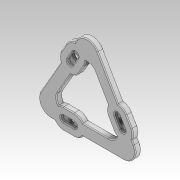
# Autodesk Inventor part: ValveThing2
Saved by Autodesk Inventor 2020 (Build 240168000, 168)
## iProperties
Created: 2022-01-09
Part Number: ValveThing2
Material: Generic
Document SubType Name: Modeling
Designer: DDeGo
Density: 1 g/cm^3
Appearance: Default
Author: DDeGo
Autodesk Inventor part; units mm, degrees
ref_plane "YZ Plane" through (0, 0, 0) normal (1, 0, 0) x (0, 1, 0)
ref_plane "XZ Plane" through (0, 0, 0) normal (0, 1, 0) x (-1, 0, 0)
ref_plane "XY Plane" through (0, 0, 0) normal (0, 0, 1) x (1, 0, 0)
sketch "Block1" plane through (0, 0, 0) normal (0, 0, 1) x (1, 0, 0)
  circle A0 centre (-3.875, 6.7117) radius 2.6
  arc A1 (-0.9902, 6.6954) -> (-5.6639, 8.975) centre (-3.327, 7.8352) ccw
  line L0 (-0.9902, 6.6954) -> (-1.5381, 5.5719)
  line L1 (-6.2119, 7.8515) -> (-5.6639, 8.975)
  line L2 (-1.5381, 5.5719) -> (-2.0861, 4.4484)
  arc A2 (-1.5381, 5.5719) -> (-6.2119, 7.8515) centre (-3.875, 6.7117) ccw
  circle A3 centre (-3.875, 6.7117) radius 1.25
  line L3 (-6.7598, 6.728) -> (-6.2119, 7.8515)
  arc A4 (-6.2119, 7.8515) -> (-1.5381, 5.5719) centre (-3.875, 6.7117) ccw
  arc A5 (-6.7598, 6.728) -> (-2.0861, 4.4484) centre (-4.423, 5.5882) ccw
  line L4 (4.6199, 1.9581) -> (1.25, 6.9542)
  line L5 (1.8, 11.5037) -> (7.107, 3.6357)
  line L6 (-5.3033, -4.2052) -> (-4.0564, -4.118)
  line L7 (-3.6936, -9.3054) -> (-4.9406, -9.3926)
  arc A6 (-4.0564, -4.118) -> (-3.6936, -9.3054) centre (-3.875, -6.7117) ccw
  line L8 (-4.0564, -4.118) -> (-2.8094, -4.0308)
  circle A7 centre (-3.875, -6.7117) radius 1.25
  circle A8 centre (-3.875, -6.7117) radius 2.6
  line L9 (-2.4467, -9.2182) -> (-3.6936, -9.3054)
  arc A9 (-3.6936, -9.3054) -> (-4.0564, -4.118) centre (-3.875, -6.7117) ccw
  arc A10 (-2.4467, -9.2182) -> (-2.8094, -4.0308) centre (-2.628, -6.6245) ccw
  arc A11 (-0.4049, -7.9727) -> (-0.6142, -4.98) centre (-2.628, -6.6245) ccw
  arc A12 (-6.6475, -2.3946) -> (-6.4003, -4.5348) centre (-4.8499, -3.2713) ccw
  line L10 (-4.0057, 3.0219) -> (-6.6475, -2.3946)
  line L11 (-10.8625, -4.193) -> (-6.7021, 4.337)
  arc A13 (-6.7021, 4.337) -> (-4.0057, 3.0219) centre (-4.423, 5.5882) ccw
  arc A14 (9.2065, 2.4902) -> (4.8955, -0.4176) centre (7.051, 1.0363) ccw
  line L12 (5.5945, -1.4539) -> (4.8955, -0.4176)
  line L13 (9.2065, 2.4902) -> (9.9055, 1.4539)
  circle A15 centre (7.75, 0) radius 1.25
  line L14 (9.9055, 1.4539) -> (10.6045, 0.4176)
  arc A16 (9.9055, 1.4539) -> (5.5945, -1.4539) centre (7.75, 0) ccw
  circle A17 centre (7.75, 0) radius 2.6
  arc A18 (5.5945, -1.4539) -> (9.9055, 1.4539) centre (7.75, 0) ccw
  arc A19 (6.2935, -2.4902) -> (10.6045, 0.4176) centre (8.449, -1.0363) ccw
  arc A20 (7.1274, -3.2754) -> (10.8801, -1.9581) centre (8.449, -1.0363) ccw
  line L15 (10.8801, -1.9581) -> (11.3403, -2.6404)
  arc A21 (7.107, 3.6357) -> (4.6199, 1.9581) centre (7.051, 1.0363) ccw
  arc A22 (9.0625, -7.3107) -> (11.3403, -2.6404) centre (8.8532, -4.318) ccw
  arc A23 (5.3975, -4.5596) -> (7.1274, -3.2754) centre (5.258, -2.5645) ccw
  line L16 (9.0625, -7.3107) -> (-0.4049, -7.9727)
  line L17 (-0.6142, -4.98) -> (5.3975, -4.5596)
  line L18 (6.2935, -2.4902) -> (5.5945, -1.4539)
  arc A24 (-5.3033, -4.2052) -> (-4.9406, -9.3926) centre (-5.122, -6.7989) ccw
  arc A25 (-6.4003, -4.5348) -> (-7.1358, -8.4434) centre (-5.122, -6.7989) ccw
  line L19 (-7.1358, -8.4434) -> (-7.9568, -8.5008)
  arc A26 (-10.8625, -4.193) -> (-7.9568, -8.5008) centre (-8.1661, -5.5081) ccw
  arc A27 (-0.7272, 7.8102) -> (-3.7443, 10.4015) centre (-3.327, 7.8352) ccw
  line L20 (-3.7443, 10.4015) -> (-3.3835, 11.1412)
  arc A28 (1.25, 6.9542) -> (-0.7272, 7.8102) centre (-0.4081, 5.8358) ccw
  arc A29 (1.8, 11.5037) -> (-3.3835, 11.1412) centre (-0.6871, 9.8261) ccw
  point P0 (0, 0)
sketch "Sketch1" plane through (0, 0, 0) normal (0, 0, 1) x (1, 0, 0)
  circle A0 centre (0, 0) radius 2.6
  arc A1 (2.8767, -0.2175) -> (-1.6267, 2.3825) centre (0.625, 1.0825) ccw
  line L0 (2.8767, -0.2175) -> (2.2517, -1.3)
  line L1 (-2.2517, 1.3) -> (-1.6267, 2.3825)
  line L2 (2.2517, -1.3) -> (1.6267, -2.3825)
  arc A2 (2.2517, -1.3) -> (-2.2517, 1.3) centre (0, 0) ccw
  circle A3 centre (0, 0) radius 1.25
  line L3 (-2.8767, 0.2175) -> (-2.2517, 1.3)
  arc A4 (-2.2517, 1.3) -> (2.2517, -1.3) centre (0, 0) ccw
  arc A5 (-2.8767, 0.2175) -> (1.6267, -2.3825) centre (-0.625, -1.0825) ccw
  line L4 (8.1426, -5.3346) -> (5.1294, -0.1156)
  line L5 (5.9955, 4.3844) -> (10.7407, -3.8346)
  line L6 (-2.1864, -10.7907) -> (-0.9364, -10.7907)
  line L7 (-0.9364, -15.9907) -> (-2.1864, -15.9907)
  arc A6 (-0.9364, -10.7907) -> (-0.9364, -15.9907) centre (-0.9364, -13.3907) ccw
  line L8 (-0.9364, -10.7907) -> (0.3136, -10.7907)
  circle A7 centre (-0.9364, -13.3907) radius 1.25
  circle A8 centre (-0.9364, -13.3907) radius 2.6
  line L9 (0.3136, -15.9907) -> (-0.9364, -15.9907)
  arc A9 (-0.9364, -15.9907) -> (-0.9364, -10.7907) centre (-0.9364, -13.3907) ccw
  arc A10 (0.3136, -15.9907) -> (0.3136, -10.7907) centre (0.3136, -13.3907) ccw
  arc A11 (2.4373, -14.8907) -> (2.4373, -11.8907) centre (0.3136, -13.3907) ccw
  arc A12 (-3.401, -8.8907) -> (-3.3036, -11.043) centre (-1.6689, -9.8907) ccw
  line L10 (-0.3878, -3.6717) -> (-3.401, -8.8907)
  line L11 (-7.7311, -10.3907) -> (-2.9859, -2.1717)
  arc A13 (-2.9859, -2.1717) -> (-0.3878, -3.6717) centre (-0.625, -1.0825) ccw
  arc A14 (12.7552, -5.1237) -> (8.2518, -7.7237) centre (10.5035, -6.4237) ccw
  line L12 (8.8768, -8.8063) -> (8.2518, -7.7237)
  line L13 (12.7552, -5.1237) -> (13.3802, -6.2063)
  circle A15 centre (11.1285, -7.5063) radius 1.25
  line L14 (13.3802, -6.2063) -> (14.0052, -7.2888)
  arc A16 (13.3802, -6.2063) -> (8.8768, -8.8063) centre (11.1285, -7.5063) ccw
  circle A17 centre (11.1285, -7.5063) radius 2.6
  arc A18 (8.8768, -8.8063) -> (13.3802, -6.2063) centre (11.1285, -7.5063) ccw
  arc A19 (9.5018, -9.8888) -> (14.0052, -7.2888) centre (11.7535, -8.5888) ccw
  arc A20 (10.279, -10.7302) -> (14.1144, -9.678) centre (11.7535, -8.5888) ccw
  line L15 (14.1144, -9.678) -> (14.5259, -10.3907)
  arc A21 (10.7407, -3.8346) -> (8.1426, -5.3346) centre (10.5035, -6.4237) ccw
  arc A22 (11.9278, -14.8907) -> (14.5259, -10.3907) centre (11.9278, -11.8907) ccw
  arc A23 (8.4637, -11.8907) -> (10.279, -10.7302) centre (8.4637, -9.8907) ccw
  line L16 (11.9278, -14.8907) -> (2.4373, -14.8907)
  line L17 (2.4373, -11.8907) -> (8.4637, -11.8907)
  line L18 (9.5018, -9.8888) -> (8.8768, -8.8063)
  arc A24 (-2.1864, -10.7907) -> (-2.1864, -15.9907) centre (-2.1864, -13.3907) ccw
  arc A25 (-3.3036, -11.043) -> (-4.31, -14.8907) centre (-2.1864, -13.3907) ccw
  line L19 (-4.31, -14.8907) -> (-5.133, -14.8907)
  arc A26 (-7.7311, -10.3907) -> (-5.133, -14.8907) centre (-5.133, -11.8907) ccw
  arc A27 (3.2168, 0.8763) -> (0.3878, 3.6717) centre (0.625, 1.0825) ccw
  line L20 (0.3878, 3.6717) -> (0.7993, 4.3844)
  arc A28 (5.1294, -0.1156) -> (3.2168, 0.8763) centre (3.3974, -1.1156) ccw
  arc A29 (5.9955, 4.3844) -> (0.7993, 4.3844) centre (3.3974, 2.8844) ccw
  point P0 (0, 0)
  point P1 (0, 0)
  point P2 (-2.2517, 1.3)
  point P3 (-2.9859, -2.1717)
  point P4 (-4.31, -14.8907)
  point P5 (-0.9364, -15.9907)
  point P6 (2.4373, -14.8907)
  point P7 (13.3802, -6.2063)
  point P8 (0.3878, 3.6717)
  point P9 (3.2168, 0.8763)
  point P10 (8.8768, -8.8063)
  point P11 (2.4373, -11.8907)
  point P12 (-0.9364, -10.7907)
  point P13 (-3.3036, -11.043)
  constraints: 2 other
extrude "Extrusion1" add sketch "Sketch1" along normal blind 1.4 contours A0 | A0 L1 A1 L0 | A0 L2 A5 L3 | L20 A29 L5 A14 L4 A28 A1 | A5 L10 A12 A24 L19 A26 L11 | A14 L13 A16 L12 | A24 L6 A6 L7 | A16 A17 | A17 L14 A19 L18 | A8 A6 | L8 A10 L9 A8 | A19 L15 A22 L16 A10 L17 A23 | A3 | A7 | A15
sketch "Sketch2" plane through (0, 0, 1.4) normal (0, 0, 1) x (1, 0, 0)
  arc A0 (2.4373, -11.8907) -> (0.3136, -10.7907) centre (0.3136, -13.3907) ccw projected
  arc A1 (-2.1864, -10.7907) -> (-3.3036, -11.043) centre (-2.1864, -13.3907) ccw projected
  line L0 (0.3136, -13.3907) -> (-2.1864, -13.3907) construction
  line L1 (0.3136, -14.0907) -> (-2.1864, -14.0907)
  line L2 (-2.1864, -12.6907) -> (0.3136, -12.6907)
  arc A2 (0.3136, -14.0907) -> (0.3136, -12.6907) centre (0.3136, -13.3907) ccw
  arc A3 (-2.1864, -12.6907) -> (-2.1864, -14.0907) centre (-2.1864, -13.3907) ccw
  arc A4 (8.1426, -5.3346) -> (8.2518, -7.7237) centre (10.5035, -6.4237) ccw projected
  arc A5 (9.5018, -9.8888) -> (10.279, -10.7302) centre (11.7535, -8.5888) ccw projected
  line L3 (10.5035, -6.4237) -> (11.7535, -8.5888) construction
  line L4 (9.8973, -6.7737) -> (11.1473, -8.9388)
  line L5 (12.3597, -8.2388) -> (11.1097, -6.0737)
  arc A6 (11.1097, -6.0737) -> (9.8973, -6.7737) centre (10.5035, -6.4237) ccw
  arc A7 (11.1473, -8.9388) -> (12.3597, -8.2388) centre (11.7535, -8.5888) ccw
  arc A8 (-0.3878, -3.6717) -> (1.6267, -2.3825) centre (-0.625, -1.0825) ccw projected
  arc A9 (2.8767, -0.2175) -> (3.2168, 0.8763) centre (0.625, 1.0825) ccw projected
  line L6 (-0.625, -1.0825) -> (0.625, 1.0825) construction
  line L7 (-1.2312, -0.7325) -> (0.0188, 1.4325)
  line L8 (1.2312, 0.7325) -> (-0.0188, -1.4325)
  arc A10 (-1.2312, -0.7325) -> (-0.0188, -1.4325) centre (-0.625, -1.0825) ccw
  arc A11 (1.2312, 0.7325) -> (0.0188, 1.4325) centre (0.625, 1.0825) ccw
  point P0 (0, 0)
  point P1 (-0.9364, -13.3907)
  point P2 (11.1285, -7.5063)
  point P3 (0, 0)
  dimension "d2" = 0.7
  constraints: 24 end point, 12 point on circle, 12 tangent, 6 centre point, 3 midpoint, 3 parallel, 2 equal radius, 1 horizontal
  measures "d2" radius of A10
extrude "Extrusion2" cut sketch "Sketch2" against normal blind 0.65
sketch "Sketch3" plane through (0, 0, 1.4) normal (0, 0, 1) x (1, 0, 0)
  arc A0 (-1.2312, -0.7325) -> (-0.0188, -1.4325) centre (-0.625, -1.0825) ccw construction
  arc A1 (1.2312, 0.7325) -> (0.0188, 1.4325) centre (0.625, 1.0825) ccw construction
  line L0 (-0.625, -1.0825) -> (0.625, 1.0825) construction
  arc A2 (11.1097, -6.0737) -> (9.8973, -6.7737) centre (10.5035, -6.4237) ccw construction
  arc A3 (11.1473, -8.9388) -> (12.3597, -8.2388) centre (11.7535, -8.5888) ccw construction
  line L1 (10.5035, -6.4237) -> (11.7535, -8.5888) construction
  arc A4 (0.3136, -14.0907) -> (0.3136, -12.6907) centre (0.3136, -13.3907) ccw construction
  arc A5 (-2.1864, -12.6907) -> (-2.1864, -14.0907) centre (-2.1864, -13.3907) ccw construction
  line L2 (0.3136, -13.3907) -> (-2.1864, -13.3907) construction
  circle A6 centre (0, 0) radius 0.7
  circle A7 centre (11.1285, -7.5063) radius 0.7
  circle A8 centre (-0.9364, -13.3907) radius 0.7
  dimension "d5" = 1.4
  constraints: 6 end point, 3 centre point, 2 equal radius, 2 midpoint, 1 coincident, 1 horizontal
  measures "d5" diameter of A6
extrude "Extrusion3" cut sketch "Sketch3" against normal through all
sketch "Sketch4" plane through (0, 0, 1.4) normal (0, 0, 1) x (1, 0, 0)
  arc A0 (-2.1864, -12.6907) -> (-2.1864, -14.0907) centre (-2.1864, -13.3907) ccw construction
  line L0 (-2.1864, -12.6907) -> (0.3136, -12.6907) construction
  arc A1 (0.3136, -14.0907) -> (0.3136, -12.6907) centre (0.3136, -13.3907) ccw construction
  line L1 (0.3136, -14.0907) -> (-2.1864, -14.0907) construction
  line L2 (11.1473, -8.9388) -> (9.8973, -6.7737) construction
  arc A2 (11.1097, -6.0737) -> (9.8973, -6.7737) centre (10.5035, -6.4237) ccw construction
  line L3 (11.1097, -6.0737) -> (12.3597, -8.2388) construction
  arc A3 (11.1473, -8.9388) -> (12.3597, -8.2388) centre (11.7535, -8.5888) ccw construction
  line L4 (-1.2312, -0.7325) -> (0.0188, 1.4325) construction
  arc A4 (1.2312, 0.7325) -> (0.0188, 1.4325) centre (0.625, 1.0825) ccw construction
  line L5 (1.2312, 0.7325) -> (-0.0188, -1.4325) construction
  arc A5 (-1.2312, -0.7325) -> (-0.0188, -1.4325) centre (-0.625, -1.0825) ccw construction
  line L6 (14.0052, -7.2888) -> (12.7552, -5.1237) projected
  arc A6 (12.7552, -5.1237) -> (10.7407, -3.8346) centre (10.5035, -6.4237) ccw projected
  line L7 (10.7407, -3.8346) -> (5.9955, 4.3844) projected
  arc A7 (5.9955, 4.3844) -> (0.7993, 4.3844) centre (3.3974, 2.8844) ccw projected
  line L8 (0.7993, 4.3844) -> (0.3878, 3.6717) projected
  arc A8 (0.3878, 3.6717) -> (-1.6267, 2.3825) centre (0.625, 1.0825) ccw projected
  line L9 (-1.6267, 2.3825) -> (-2.8767, 0.2175) projected
  arc A9 (-2.8767, 0.2175) -> (-2.9859, -2.1717) centre (-0.625, -1.0825) ccw projected
  line L10 (-2.9859, -2.1717) -> (-7.7311, -10.3907) projected
  arc A10 (-7.7311, -10.3907) -> (-5.133, -14.8907) centre (-5.133, -11.8907) ccw projected
  line L11 (-5.133, -14.8907) -> (-4.31, -14.8907) projected
  arc A11 (-4.31, -14.8907) -> (-2.1864, -15.9907) centre (-2.1864, -13.3907) ccw projected
  line L12 (-2.1864, -15.9907) -> (0.3136, -15.9907) projected
  arc A12 (0.3136, -15.9907) -> (2.4373, -14.8907) centre (0.3136, -13.3907) ccw projected
  line L13 (2.4373, -14.8907) -> (11.9278, -14.8907) projected
  arc A13 (11.9278, -14.8907) -> (14.5259, -10.3907) centre (11.9278, -11.8907) ccw projected
  line L14 (14.5259, -10.3907) -> (14.1144, -9.678) projected
  arc A14 (14.1144, -9.678) -> (14.0052, -7.2888) centre (11.7535, -8.5888) ccw projected
  arc A15 (2.4373, -11.8907) -> (0.3136, -10.7907) centre (0.3136, -13.3907) ccw projected
  line L15 (0.3136, -10.7907) -> (-2.1864, -10.7907) projected
  arc A16 (-2.1864, -10.7907) -> (-3.3036, -11.043) centre (-2.1864, -13.3907) ccw projected
  arc A17 (-3.401, -8.8907) -> (-3.3036, -11.043) centre (-1.6689, -9.8907) ccw projected
  line L16 (-3.401, -8.8907) -> (-0.3878, -3.6717) projected
  arc A18 (-0.3878, -3.6717) -> (1.6267, -2.3825) centre (-0.625, -1.0825) ccw projected
  line L17 (1.6267, -2.3825) -> (2.8767, -0.2175) projected
  arc A19 (2.8767, -0.2175) -> (3.2168, 0.8763) centre (0.625, 1.0825) ccw projected
  arc A20 (5.1294, -0.1156) -> (3.2168, 0.8763) centre (3.3974, -1.1156) ccw projected
  line L18 (5.1294, -0.1156) -> (8.1426, -5.3346) projected
  arc A21 (8.1426, -5.3346) -> (8.2518, -7.7237) centre (10.5035, -6.4237) ccw projected
  line L19 (8.2518, -7.7237) -> (9.5018, -9.8888) projected
  arc A22 (9.5018, -9.8888) -> (10.279, -10.7302) centre (11.7535, -8.5888) ccw projected
  arc A23 (8.4637, -11.8907) -> (10.279, -10.7302) centre (8.4637, -9.8907) ccw projected
  line L20 (8.4637, -11.8907) -> (2.4373, -11.8907) projected
  arc A24 (0.4781, 3.5281) -> (-1.4968, 2.3075) centre (0.625, 1.0825) ccw
  line L21 (0.4781, 3.5281) -> (0.9292, 4.3094)
  arc A25 (5.8655, 4.3094) -> (0.9292, 4.3094) centre (3.3974, 2.8844) ccw
  line L22 (5.8655, 4.3094) -> (10.6504, -3.9781)
  arc A26 (12.6253, -5.1987) -> (10.6504, -3.9781) centre (10.5035, -6.4237) ccw
  line L23 (12.6253, -5.1987) -> (13.8753, -7.3638)
  arc A27 (13.9449, -9.6844) -> (13.8753, -7.3638) centre (11.7535, -8.5888) ccw
  line L24 (13.9449, -9.6844) -> (14.396, -10.4657)
  arc A28 (11.9278, -14.7407) -> (14.396, -10.4657) centre (11.9278, -11.8907) ccw
  line L25 (11.9278, -14.7407) -> (2.3581, -14.7407)
  arc A29 (0.3136, -15.8407) -> (2.3581, -14.7407) centre (0.3136, -13.3907) ccw
  line L26 (0.3136, -15.8407) -> (-2.1864, -15.8407)
  arc A30 (-4.2309, -14.7407) -> (-2.1864, -15.8407) centre (-2.1864, -13.3907) ccw
  line L27 (-4.2309, -14.7407) -> (-5.133, -14.7407)
  arc A31 (-7.6012, -10.4657) -> (-5.133, -14.7407) centre (-5.133, -11.8907) ccw
  line L28 (-7.6012, -10.4657) -> (-2.8164, -2.1781)
  arc A32 (-2.7468, 0.1425) -> (-2.8164, -2.1781) centre (-0.625, -1.0825) ccw
  line L29 (-2.7468, 0.1425) -> (-1.4968, 2.3075)
  line L30 (-0.4781, -3.5281) -> (-3.5309, -8.8157)
  arc A33 (-3.5309, -8.8157) -> (-3.348, -11.2336) centre (-1.6689, -9.8907) ccw
  arc A34 (-2.1864, -10.9407) -> (-3.348, -11.2336) centre (-2.1864, -13.3907) ccw
  line L31 (-2.1864, -10.9407) -> (0.3136, -10.9407)
  arc A35 (2.3581, -12.0407) -> (0.3136, -10.9407) centre (0.3136, -13.3907) ccw
  line L32 (2.3581, -12.0407) -> (8.4637, -12.0407)
  arc A36 (8.4637, -12.0407) -> (10.4662, -10.6733) centre (8.4637, -9.8907) ccw
  arc A37 (9.6317, -9.8138) -> (10.4662, -10.6733) centre (11.7535, -8.5888) ccw
  line L33 (9.6317, -9.8138) -> (8.3817, -7.6487)
  arc A38 (8.3121, -5.3281) -> (8.3817, -7.6487) centre (10.5035, -6.4237) ccw
  line L34 (8.3121, -5.3281) -> (5.2593, -0.0406)
  arc A39 (5.2593, -0.0406) -> (3.0739, 1.01) centre (3.3974, -1.1156) ccw
  arc A40 (2.7468, -0.1425) -> (3.0739, 1.01) centre (0.625, 1.0825) ccw
  line L35 (2.7468, -0.1425) -> (1.4968, -2.3075)
  arc A41 (-0.4781, -3.5281) -> (1.4968, -2.3075) centre (-0.625, -1.0825) ccw
  point P0 (0, 0)
  dimension "d10" = 0.15
  dimension "d13" = 0.15
  constraints: 36 point on circle, 30 end point, 18 centre point, 31 other
  measures "d10" distance between parallel lines of L9 L29
  measures "d13" distance between parallel lines of L17 L35
extrude "Extrusion4" cut sketch "Sketch4" against normal through all
fillet "Fillet1" radius 0.2 66 edges at (-3.8128, -10.0529, 1.4) (-2.0045, -6.1719, 1.4) (-7.6012, -13.3157, 1.4) (-4.682, -14.7407, 1.4) (-5.2088, -6.3219, 1.4) (-2.1218, 1.225, 1.4) (-0.6631, 3.1666, 1.4) (-3.0739, -1.0091, 1.4) (2.1218, -1.225, 1.4) (2.9819, 0.4134, 1.4) (0.6631, -3.1666, 1.4) (2.1218, -1.225, 0) (2.9819, 0.4134, 0) (0.6631, -3.1666, 0) (-3.8128, -10.0529, 0) (-2.0045, -6.1719, 0) (-7.6012, -13.3157, 0) (-4.682, -14.7407, 0) (-5.2088, -6.3219, 0) (0.7037, 3.9188, 1.4) (8.258, 0.1656, 1.4) (3.3974, 5.7344, 1.4) (8.258, 0.1656, 0) (0.7037, 3.9188, 0) (3.3974, 5.7344, 0) (-2.1218, 1.225, 0) (-3.0739, -1.0091, 0) (-0.6631, 3.1666, 0) (6.7857, -2.6844, 0) (4.3289, 0.8222, 0) (6.7857, -2.6844, 1.4) (4.3289, 0.8222, 1.4) (9.0067, -8.7313, 1.4) (8.0546, -6.4972, 1.4) (9.9956, -10.2954, 1.4) (8.0546, -6.4972, 0) (9.9956, -10.2954, 0) (9.0067, -8.7313, 0) (13.2503, -6.2813, 1.4) (11.7916, -4.3397, 1.4) (14.2024, -8.5153, 1.4) (13.2503, -6.2813, 0) (11.7916, -4.3397, 0) (14.2024, -8.5153, 0) (7.143, -14.7407, 0) (14.1704, -10.075, 0) (14.396, -13.3157, 0) (14.1704, -10.075, 1.4) (7.143, -14.7407, 1.4) (14.396, -13.3157, 1.4) (5.4109, -12.0407, 0) (9.6761, -11.6663, 0) (5.4109, -12.0407, 1.4) (9.6761, -11.6663, 1.4) (-0.9364, -10.9407, 1.4) (-2.7854, -11.015, 1.4) (1.4745, -11.2332, 1.4) (-0.9364, -10.9407, 0) (-2.7854, -11.015, 0) (1.4745, -11.2332, 0) (-0.9364, -15.8407, 0) (-3.3472, -15.5482, 0) (1.4745, -15.5482, 0) (-0.9364, -15.8407, 1.4) (-3.3472, -15.5482, 1.4) (1.4745, -15.5482, 1.4)
fillet "Fillet2" radius 0.2 15 edges at (-0.6062, 0.35, 1.4) (0.975, 1.6887, 1.4) (0.6062, -0.35, 1.4) (-0.975, -1.6887, 1.4) (-2.8864, -13.3907, 1.4) (-0.9364, -12.6907, 1.4) (1.0136, -13.3907, 1.4) (-0.9364, -14.0907, 1.4) (12.1035, -9.195, 1.4) (10.5223, -7.8563, 1.4) (10.1535, -5.8175, 1.4) (11.7347, -7.1563, 1.4) (10.4285, -7.5063, 0) (-1.6364, -13.3907, 0) (-0.7, 0, 0)
equation "\"d13\" = d10"
body "Solid1"
